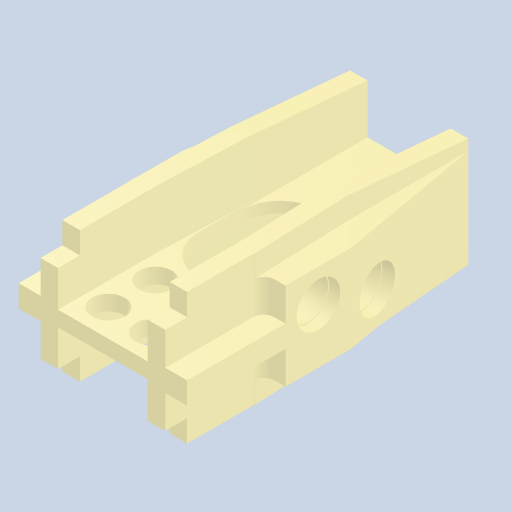
# Autodesk Inventor part: Payload_CommercialNP2_Short
Saved by Autodesk Inventor 2023 (Build 270158000, 158)
## iProperties
Created: 2021-05-04
Part Number: Payload_CommercialNP2_Short
Material: Nylon 6/6
Document SubType Name: Modeling
Designer: Pip
Density: 1.13 g/cm^3
Appearance: Snow
Mass: 0.292863 g
Surface Area: 7.23197 cm^2
Volume: 0.25917 cm^3
InterProbeDist: 2.000 mm
WallThickness: 0.800 mm
Author: Pip
Autodesk Inventor part; units mm, degrees
ref_plane "YZ Plane" through (0, 0, 0) normal (1, 0, 0) x (0, 1, 0)
ref_plane "XZ Plane" through (0, 0, 0) normal (0, 1, 0) x (-1, 0, 0)
ref_plane "XY Plane" through (0, 0, 0) normal (0, 0, 1) x (1, 0, 0)
sketch "Sk:Base" plane through (0, 0, 0) normal (0, 1, 0) x (-1, 0, 0)
  line L0 (0, -2.25) -> (-2.05, -2.25)
  line L1 (-2.05, -2.25) -> (-2.05, 2.25)
  line L2 (-2.05, 2.25) -> (0, 2.25)
  line L3 (0, 2.25) -> (0, -2.25)
  line L4 (-2.05, -2.25) -> (-1.9, -6.25)
  line L5 (-1.9, -6.25) -> (0, -6.25)
  line L6 (0, -6.25) -> (0, -2.25)
  line L7 (-2.05, 2.25) -> (-2.85, 2.25)
  line L8 (-2.85, -2.25) -> (-2.05, -2.25)
  line L9 (-2.05, -2.25) -> (-2.05, 2.25)
  line L10 (-2.7, -6.25) -> (-1.9, -6.25)
  line L11 (0, 2.25) -> (-2.5, 2.25)
  line L12 (-2.85, -2.25) -> (-2.85, 2.25)
  line L13 (-2.85, -2.25) -> (-2.7, -6.25)
  line L14 (-1.9, -6.25) -> (-1.9, -2.25)
  line L15 (-3.85, -2.25) -> (-2.85, -2.25)
  line L16 (-3.85, -2.25) -> (-3.85, -5.228)
  line L17 (-2.85, 2.25) -> (-3.85, 2.25)
  line L18 (-3.85, 2.25) -> (-3.85, -2.25)
  line L19 (-3.85, -2.25) -> (-2.85, -2.25)
  line L20 (-2.85, -2.25) -> (-2.85, 2.25)
  line L21 (-2.7, -6.25) -> (-1.9, -6.25)
  line L22 (-1.9, -6.25) -> (-1.9, -11.75)
  line L23 (-1.9, -11.75) -> (-2.7, -11.75)
  line L24 (-2.7, -11.75) -> (-2.7, -6.25)
  line L25 (-1.9, -11.75) -> (0, -11.75)
  line L26 (0, -11.75) -> (0, -7.75)
  line L27 (0, -7.75) -> (-1.9, -7.75)
  line L28 (-1.9, -7.75) -> (-1.9, -11.75)
  line L29 (-2.7, -11.75) -> (-3.85, -5.228)
  line L30 (-0.3, -8.25) -> (-0.3, -11.25)
  line L31 (-0.5, -11.45) -> (-1.4, -11.45)
  line L32 (-1.6, -11.25) -> (-1.6, -8.25)
  line L33 (-1.4, -8.05) -> (-0.5, -8.05)
  arc A0 (-0.3, -8.25) -> (-0.5, -8.05) centre (-0.5, -8.25) ccw
  arc A1 (-1.4, -8.05) -> (-1.6, -8.25) centre (-1.4, -8.25) ccw
  arc A2 (-1.6, -11.25) -> (-1.4, -11.45) centre (-1.4, -11.25) ccw
  arc A3 (-0.5, -11.45) -> (-0.3, -11.25) centre (-0.5, -11.25) ccw
  point P0 (0, 0)
  point P1 (-2.85, -2.25)
  point P2 (-1.9, -7.75)
  point P3 (-3.35, -2.25)
  point P4 (-0.3, -8.05)
  point P5 (-0.3, -11.45)
  point P6 (-1.6, -11.45)
  point P7 (-1.6, -8.05)
  dimension "d4" = 2.05
  dimension "d3" = 4.5
  dimension "d5" = 0
  dimension "d6" = 1.9
  dimension "d7" = 0
  dimension "d1" = 0.8
  dimension "d40" = 2.25
  dimension "d41" = 4
  dimension "d148" = 4.5
  dimension "d167" = 5.5
  dimension "d168" = 0.8
  dimension "d169" = 4
  dimension "d172" = 1
  dimension "d173" = 1
  dimension "d232" = 10
  dimension "d289" = 2.05
  dimension "d293" = 0
  dimension "d307" = 0.3
  dimension "d310" = 0.2
  constraints: 68 end point, 13 parallel, 11 point on line, 8 horizontal, 8 point on circle, 8 tangent, 6 perpendicular, 4 centre point, 3 equal radius, 3 vertical, 1 midpoint, 3 other
  measures "d4" distance of L0.start L0.end
  measures "d3" distance of L0.end L1.end
  measures "d5" distance from line of point (0, 0) L3
  measures "d6" distance of L4.end L5.end
  measures "d7" horizontal distance of L0.start L5.end
  measures "d1" distance between parallel lines of L12 L1
  measures "d40" distance from line of point (0, 0) L2
  measures "d41" distance between parallel lines of L0 L5
  measures "d148" distance of L17.end L18.end
  measures "d167" distance of L21.end L22.end
  measures "d168" distance between parallel lines of L24 L22
  measures "d169" distance of L26.end L25.end
  measures "d172" distance between parallel lines of L12 L18
  measures "d173" distance between parallel lines of L12 L16
  measures "d232" angle of L24 L29
  measures "d289" distance between parallel lines of L1 L26
  measures "d293" distance from line of point (-3.35, -2.25) L15
  measures "d307" distance between parallel lines of L26 L30
  measures "d310" radius of A0
extrude "Ex:Midline" add sketch "Sk:Base" along normal blind 0.35 contours L0 L1 L2 L3 | L14 L4 L0
extrude "Ex:FrontSupport" add sketch "Sk:Base" along normal blind 0.25 contours L27 L26 L25 L22 | L30 A3 L31 A2 L32 A1 L33 A0
extrude "Ex:SideRidge" add sketch "Sk:Base" along normal blind 0.5 contours L15 L18 L17 L12
extrude "Ex:SideWall" add sketch "Sk:Base" along normal blind 3 contours L8 L12 L7 L1 | L4 L10 L13 L8 | L22 L23 L24 L10
sketch "Sk:BaseHole" plane through (0, 0.35, 0) normal (0, 1, 0) x (1, 0, 0)
  circle A0 centre (1, -1) radius 0.75
  line L0 (0, -2.25) -> (2.05, -2.25) projected
  line L1 (0, 2.25) -> (0, -2.25) projected
  point P0 (0, 0)
  dimension "d68" = 1.5
  dimension "d69" = 1.25
  dimension "d79" = 1
  constraints: 1 centre point
  measures "d68" diameter of A0
  measures "d69" distance from line of A0.centre L0
  measures "d79" distance from line of A0.centre L1
extrude "Ex:BaseHole" cut sketch "Sk:BaseHole" along normal through all both and the other way through all
pattern_linear "Pat:BaseHoles" count 4 spacing 2.15 along (0, 0, -1) of "Ex:BaseHole"
extrude "Ex:RemMaterial" [suppressed]
fillet "Fillet:Support" radius 1.75 2 edges at (1.9, 0.175, -2.25) (1.9, 0.125, -7.75)
extrude "Ex:Widening" add sketch "Sk:Base" along normal blind 2 contours L22 L23 L24 L10 | L13 L24 L29 L16 L15
fillet "Fillet:Side" radius 0.5 1 edges at (2.85, 1.25, -2.25)
sketch "Sk:FrontTaper" plane through (2.7, 3, -6.25) normal (1, 0, 0) x (0, 0, -1)
  line L0 (5.5, 0) -> (0, 0) projected
  line L1 (0, -1) -> (5.5, -1) projected
  line L2 (0, 0) -> (5.5, 0)
  line L3 (5.5, 0) -> (5.5, -1)
  line L4 (5.5, -1) -> (0, -1)
  line L5 (0, -1) -> (0, 0)
  line L6 (0, 0) -> (-4, 0) projected
  line L7 (0, 0) -> (5.5, -0.5)
  point P0 (-6.25, -3)
  point P1 (5.5, -0.5)
  point P2 (4.5, 0)
  dimension "d219" = 1
  dimension "d222" = 0.5
  dimension "d223" = 0
  constraints: 10 end point, 2 parallel, 1 horizontal, 1 perpendicular
  measures "d219" distance of L4.end L0.end
  measures "d222" distance of L0.start L7.end
  measures "d223" distance from line of L3 L7.end
extrude "Ex:FrontTaper" cut sketch "Sk:FrontTaper" against normal up to next contours L3 L7 L0
sketch "Sk:LidNotch" plane through (2.85, 0.5, 2.25) normal (1, 0, 0) x (0, 0, -1)
  line L0 (0, -0.15) -> (0, 2.5) projected
  line L1 (0, 2.5) -> (1, 2.5)
  line L2 (1, 2.5) -> (1, 1.5)
  line L3 (1, 1.5) -> (0, 1.5)
  line L4 (0, 1.5) -> (0, 2.5)
  line L5 (0, 2.5) -> (4.5, 2.5) projected
  point P0 (2.25, -0.5)
  point P1 (0, 1.5)
  dimension "d224" = 1
  dimension "d225" = 1
  constraints: 8 end point, 2 parallel, 1 horizontal, 1 perpendicular
  measures "d224" distance between parallel lines of L0 L2
  measures "d225" distance between parallel lines of L5 L3
extrude "Ex:LidNotch" cut sketch "Sk:LidNotch" against normal up to next
mirror "Mirror1" about plane through (0, 0, -2.25) normal (-1, 0, 0)
mirror "Mirror2" about plane through (0.95, 0, -9.75) normal (0, -1, 0)
sketch "Sk:ThreadHole1" plane through (3.85, 2, -2.25) normal (1, 0, 0) x (0, 0, -1)
  circle A0 centre (1.5, -1.5) radius 0.95
  circle A1 centre (1.5, -1.5) radius 1
  line L0 (0, 0) -> (2.978, 0) projected
  line L1 (0, -1.5) -> (0, 0) projected
  line L2 (0, -4) -> (2.978, -4) projected
  point P0 (-2.25, -2)
  dimension "d130" = 1.9
  dimension "d131" = 2
  dimension "d199" = 1.5
  dimension "d200" = 1.5
  constraints: 2 centre point, 1 concentric
  measures "d130" diameter of A0
  measures "d131" diameter of A1
  measures "d199" distance from line of L0 A0.centre
  measures "d200" distance from line of L1 A0.centre
sketch "Sk:ThreadHole2" plane through (2.7, -2, -11.75) normal (0.9848078, 0, -0.1736482) x (-0.1736482, 0, -0.9848078)
  circle A0 centre (-5.1226, 1.5) radius 1
  circle A1 centre (-5.1226, 1.5) radius 0.95
  line L0 (-6.6226, 4) -> (0, 4) projected
  line L1 (-6.6226, 0) -> (-6.6226, 4) projected
  line L2 (-6.6226, 0) -> (0, 0) projected
  point P0 (-11.1026, 2)
  dimension "d298" = 2
  dimension "d299" = 1.9
  dimension "d301" = 1.5
  dimension "d304" = 1.5
  constraints: 2 centre point, 1 coincident
  measures "d298" diameter of A0
  measures "d299" diameter of A1
  measures "d301" distance from line of L1 A0.centre
  measures "d304" distance from line of L2 A0.centre
extrude "Ex:ThreadHole1" cut sketch "Sk:ThreadHole1" against normal blind 1.5 contours A0
extrude "Ex:ThreadHole2" cut sketch "Sk:ThreadHole2" against normal blind 1.5 contours A1
extrude "Ex:ThreadEntry1" cut sketch "Sk:ThreadHole1" against normal blind 0.5 contours A0 | A1
extrude "Ex:ThreadEntry2" cut sketch "Sk:ThreadHole2" against normal blind 0.5 contours A0 | A1
pattern_circular "Pat:Threads" count 2 over 360 about axis through (0, 0, -10) along (0, 0, 1) of "Ex:ThreadEntry1", "Ex:ThreadHole1", "Ex:ThreadEntry2", "Ex:ThreadHole2"
equation "\"d40\" = 0.5 * d3"
equation "\"SideWallHeight\" = 3"
body "Solid1"
